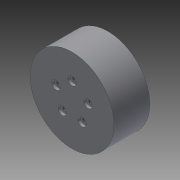
# Autodesk Inventor part: Aluminum mold support
Saved by Autodesk Inventor 2013 (Build 170138000, 138)
## iProperties
Created: 2013-05-10
Part Number: Aluminum mold support
Material: Generic
Document SubType Name: Modeling
Designer: grtstudent
Density: 1 g/cm^3
Author: grtstudent
Autodesk Inventor part; units mm, degrees
ref_plane "YZ Plane" through (0, 0, 0) normal (1, 0, 0) x (0, 1, 0)
ref_plane "XZ Plane" through (0, 0, 0) normal (0, 1, 0) x (-1, 0, 0)
ref_plane "XY Plane" through (0, 0, 0) normal (0, 0, 1) x (1, 0, 0)
sketch "Sketch1" plane through (0, 0, 0) normal (0, 0, 1) x (1, 0, 0)
  circle A0 centre (0, 0) radius 47.371
  dimension "d0" = 94.742
  constraints: 1 centre point, 1 coincident
  measures "d0" diameter of A0
extrude "Extrusion1" add sketch "Sketch1" along normal blind 40.64
sketch "Sketch2" plane through (0, 0, 0) normal (0, 0, -1) x (-1, 0, 0)
  circle A0 centre (0, 0) radius 42.8625
  dimension "d4" = 85.725
  constraints: 1 centre point, 1 coincident
  measures "d4" diameter of A0
extrude "Extrusion2" cut sketch "Sketch2" against normal blind 31.75
sketch "Sketch3" plane through (0, 0, 31.75) normal (0, 0, -1) x (-1, 0, 0)
  circle A0 centre (-11.1973, -15.4118) radius 1.905
  circle A1 centre (18.1176, 5.8868) radius 1.905
  circle A2 centre (0, 19.05) radius 1.905
  circle A3 centre (11.1973, -15.4118) radius 1.905
  circle A4 centre (-18.1176, 5.8868) radius 1.905
  circle A5 centre (0, 0) radius 42.8625
  constraints: 6 centre point
extrude "Extrusion3" cut sketch "Sketch3" against normal blind 31.75 contours A0 | A1 | A2 | A3 | A4
sketch "Sketch4" plane through (0, 0, 40.64) normal (0, 0, 1) x (1, 0, 0)
  circle A0 centre (-11.1973, -15.4118) radius 1.905 projected
  circle A1 centre (-18.1176, 5.8868) radius 1.905 projected
  circle A2 centre (11.1973, -15.4118) radius 1.905 projected
  circle A3 centre (0, 19.05) radius 1.905 projected
  circle A4 centre (18.1176, 5.8868) radius 1.905 projected
  circle A5 centre (0, 0) radius 47.371 projected
hole "Hole1" at (0, 19.05, 40.64) at (18.1176, 5.8868, 40.64) at (11.1973, -15.4118, 40.64) at (-11.1973, -15.4118, 40.64) at (-18.1176, 5.8868, 40.64) direction (0, 0, -1) diameter 9.525 depth 3.175
sketch "Sketch5" plane through (-18.1176, 5.8868, 37.465) normal (0, 0, 1) x (1, 0, 0)
  circle A0 centre (0, 0) radius 1.905 projected
  circle A1 centre (0, 0) radius 4.7625 projected
  circle A2 centre (18.1176, 13.1632) radius 1.905 projected
  circle A3 centre (36.2353, 0) radius 1.905 projected
  circle A4 centre (29.3149, -21.2985) radius 1.905 projected
  circle A5 centre (6.9203, -21.2985) radius 1.905 projected
  point P0 (18.1176, -5.8868)
hole "Hole2" at (-18.1176, 5.8868, 37.465) at (0, 19.05, 37.465) at (-11.1973, -15.4118, 37.465) at (11.1973, -15.4118, 37.465) at (18.1176, 5.8868, 37.465) direction (0, 0, -1) diameter 5.3594 depth 25.4 thread size "1/4-28 UNF" class "2B" standard "ANSI Unified Screw Threads"
body "Solid1"
